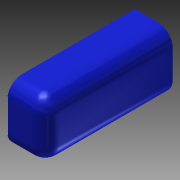
# Autodesk Inventor part: Bumper Cover Part3 (26x28 robot)
Saved by Autodesk Inventor 2014 SP1 (Build 180222100, 222)
## iProperties
Created: 2013-01-06
Part Number: Bumper Cover Part3 (26x28 robot)
Material: Generic
Document SubType Name: Modeling
Designer: Moses
Density: 1 g/cm^3
Mass: 177.489 g
Surface Area: 2179.08 cm^2
Volume: 177.489 cm^3
Appearance: Blue - Wall Paint - Glossy
Author: Moses
Autodesk Inventor part; units mm, degrees
ref_plane "YZ Plane" through (0, 0, 0) normal (1, 0, 0) x (0, 1, 0)
ref_plane "XZ Plane" through (0, 0, 0) normal (0, 1, 0) x (-1, 0, 0)
ref_plane "XY Plane" through (0, 0, 0) normal (0, 0, 1) x (1, 0, 0)
sketch "Sketch1" plane through (0, 0, 0) normal (0, 0, 1) x (1, 0, 0)
  circle A0 centre (38.1, -31.75) radius 31.75 construction
  circle A1 centre (38.1, 31.75) radius 31.75 construction
  line L0 (6.35, 63.5) -> (38.1, 63.5) construction
  line L1 (69.85, 31.75) -> (69.85, -31.75) construction
  line L2 (6.35, -63.5) -> (38.1, -63.5) construction
  line L3 (38.1, 65.0875) -> (-14.2875, 65.0875)
  line L4 (-14.2875, -65.0875) -> (38.1, -65.0875)
  arc A2 (38.1, -65.0875) -> (71.4375, -31.75) centre (38.1, -31.75) ccw
  arc A3 (71.4375, 31.75) -> (38.1, 65.0875) centre (38.1, 31.75) ccw
  line L5 (71.4375, 31.75) -> (71.4375, -31.75)
  line L6 (38.1, 65.0875) -> (38.1, 63.5) construction
  arc A4 (69.85, 31.75) -> (38.1, 63.5) centre (38.1, 31.75) ccw
  arc A5 (38.1, -63.5) -> (69.85, -31.75) centre (38.1, -31.75) ccw
  line L7 (69.85, 31.75) -> (69.85, -31.75)
  line L8 (-12.7, 63.5) -> (-12.7, 38.1)
  line L9 (-12.7, 38.1) -> (-14.2875, 38.1)
  line L10 (-14.2875, 38.1) -> (-14.2875, 65.0875)
  line L11 (-14.2875, -65.0875) -> (-14.2875, -38.1)
  line L12 (-14.2875, -38.1) -> (-12.7, -38.1)
  line L13 (-12.7, -63.5) -> (-12.7, -38.1)
  line L14 (-12.7, 38.1) -> (-12.7, -38.1)
  line L15 (-12.7, -63.5) -> (-12.7, 63.5) construction
  line L16 (-12.7, 63.5) -> (6.35, 63.5) construction
  line L17 (6.35, 63.5) -> (6.35, -63.5) construction
  line L18 (6.35, -63.5) -> (-12.7, -63.5) construction
  line L19 (-12.7, -63.5) -> (38.1, -63.5)
  line L20 (-12.7, 63.5) -> (38.1, 63.5)
  point P0 (0, 0)
  point P1 (38.1, 64.2937)
  dimension "d3" = 25.4
  dimension "d7" = 25.4
  dimension "d9" = 1.5875
  dimension "d15" = 1.5875
  dimension "d16" = 1.5875
  constraints: 34 end point, 14 tangent, 12 point on circle, 4 centre point, 4 parallel, 4 perpendicular, 2 coincident, 2 collinear, 2 point on line, 1 concentric, 1 midpoint, 1 vertical
  measures "d3" distance of L8.start L8.end
  measures "d7" distance of L13.start L12.end
  measures "d9" distance of L3.start L0.end
  measures "d15" distance of L11.end L12.end
  measures "d16" distance between parallel lines of L8 L10
extrude "Extrusion1" add sketch "Sketch1" along normal blind 1.5875
extrude "Extrusion2" add sketch "Sketch1" against normal blind 285.75 contours A3 L5 A2 L4 L11 L12 L13 L19 A5 L7 A4 L20 L8 L9 L10 L3
sketch "Sketch2" plane through (0, 0, -285.75) normal (0, 0, -1) x (-1, 0, 0)
  arc A0 (-38.1, 63.5) -> (-69.85, 31.75) centre (-38.1, 31.75) ccw projected
  line L0 (-38.1, 63.5) -> (12.7, 63.5) projected
  line L1 (12.7, 63.5) -> (12.7, 38.1) projected
  line L2 (12.7, 38.1) -> (14.2875, 38.1) projected
  line L3 (14.2875, 38.1) -> (14.2875, 65.0875) projected
  line L4 (14.2875, 65.0875) -> (-38.1, 65.0875) projected
  arc A1 (-38.1, 65.0875) -> (-71.4375, 31.75) centre (-38.1, 31.75) ccw projected
  line L5 (-71.4375, 31.75) -> (-71.4375, -31.75) projected
  arc A2 (-71.4375, -31.75) -> (-38.1, -65.0875) centre (-38.1, -31.75) ccw projected
  line L6 (-38.1, -65.0875) -> (14.2875, -65.0875) projected
  line L7 (14.2875, -65.0875) -> (14.2875, -38.1) projected
  line L8 (14.2875, -38.1) -> (12.7, -38.1) projected
  line L9 (12.7, -38.1) -> (12.7, -63.5) projected
  line L10 (12.7, -63.5) -> (-38.1, -63.5) projected
  arc A3 (-69.85, -31.75) -> (-38.1, -63.5) centre (-38.1, -31.75) ccw projected
  line L11 (-69.85, -31.75) -> (-69.85, 31.75) projected
  line L12 (12.7, -63.5) -> (12.7, 63.5) projected
extrude "Extrusion3" add sketch "Sketch2" along normal blind 1.5875
fillet "Fillet1" radius 33.3375 8 edges at (61.6732, -55.3232, 1.5875) (71.4375, 0, 1.5875) (61.6732, 55.3232, 1.5875) (11.9062, 65.0875, 1.5875) (11.9062, -65.0875, 1.5875) (60.5506, -54.2006, 0) (69.85, 0, 0) (60.5506, 54.2006, 0)
body "Solid1"
